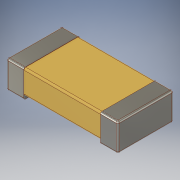
# Autodesk Inventor part: Capacitor_3216-1.6mm
Saved by Autodesk Inventor 2018 (Build 220112000, 112)
## iProperties
Created: 2016-08-15
Part Number: Capacitor_3216-1.6mm
Material: Copper
Document SubType Name: Modeling
Designer: Bradley
Density: 8.94 g/cm^3
Appearance: Copper - Satin
Author: Bradley
Autodesk Inventor part; units mm, degrees
ref_plane "YZ Plane" through (0, 0, 0) normal (1, 0, 0) x (0, 1, 0)
ref_plane "XZ Plane" through (0, 0, 0) normal (0, 1, 0) x (-1, 0, 0)
ref_plane "XY Plane" through (0, 0, 0) normal (0, 0, 1) x (1, 0, 0)
sketch "Sketch1" plane through (0, 0, 0) normal (0, 0, 1) x (1, 0, 0)
  line L0 (-1.6, 0.7) -> (-1.1, 0.7)
  line L1 (-1.1, 0.7) -> (-1.1, -0.1)
  line L2 (-1.1, -0.1) -> (-1.6, -0.1)
  line L3 (-1.6, -0.1) -> (-1.6, 0.7)
  line L4 (-1.1, 0.69) -> (1.1, 0.69)
  line L5 (1.1, 0.69) -> (1.1, 0)
  line L6 (1.1, 0) -> (-1.1, 0)
  line L7 (-1.1, 0) -> (-1.1, 0.69)
  line L8 (1.1, 0.7) -> (1.6, 0.7)
  line L9 (1.6, 0.7) -> (1.6, -0.1)
  line L10 (1.6, -0.1) -> (1.1, -0.1)
  line L11 (1.1, -0.1) -> (1.1, 0.7)
  point P0 (0, 0)
  point P1 (0, 0.69)
  point P2 (0, 0)
  dimension "d0" = 3.2
  dimension "d1" = 0.8
  dimension "d2" = 0.5
  dimension "d3" = 0.1
  dimension "d6" = 0.01
  constraints: 24 end point, 6 parallel, 3 horizontal, 3 perpendicular, 3 point on line, 2 collinear, 2 midpoint, 1 coincident, 1 vertical alignment
  measures "d0" distance between parallel lines of L9 L3
  measures "d1" distance of L2.end L0.start
  measures "d2" distance of L1.end L2.end
  measures "d3" distance between parallel lines of L2 L6
  measures "d6" distance between parallel lines of L4 L0
extrude "Extrusion1" add sketch "Sketch1" along normal mid plane 1.6 contours L0 L1 L2 L3 | L11 L8 L9 L10 L5
extrude "Extrusion2" add sketch "Sketch1" along normal mid plane 1.59 contours L4 L5 L6 L1
fillet "Fillet1" radius 0.05 20 edges at (0, 0.69, 0.795) (0, 0, 0.795) (0, 0.69, -0.795) (0, 0, -0.795) (-1.35, 0.7, 0.8) (-1.35, -0.1, 0.8) (1.35, -0.1, 0.8) (1.35, 0.7, 0.8) (1.35, 0.7, -0.8) (1.35, -0.1, -0.8) (1.6, 0.3, -0.8) (1.6, -0.1, 0) (1.6, 0.3, 0.8) (1.6, 0.7, 0) (-1.6, 0.7, 0) (-1.6, 0.3, 0.8) (-1.6, -0.1, 0) (-1.35, 0.7, -0.8) (-1.35, -0.1, -0.8) (-1.6, 0.3, -0.8)
body "Solid1"
